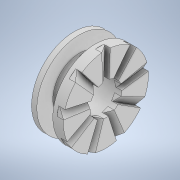
# Autodesk Inventor part: Part11
Saved by Autodesk Inventor 2021 (Build 250183000, 183)
## iProperties
Created: 2022-12-10
Part Number: Part11
Material: Generic
Document SubType Name: Modeling
Designer: user
Density: 1 g/cm^3
Appearance: Default
Author: user
Autodesk Inventor part; units mm, degrees
sketch "Sketch1" plane through (0, 0, 0) normal (0, 0, 1) x (1, 0, 0)
  line L0 (0, 0) -> (0, 40)
  line L1 (0, 40) -> (5, 40)
  line L2 (5, 40) -> (5, 15)
  line L3 (5, 25) -> (20, 25)
  line L4 (20, 15) -> (20, 40)
  line L5 (20, 40) -> (24, 40)
  line L6 (24, 40) -> (24, 0)
  line L7 (24, 0) -> (0, 0)
  line L8 (5, 15) -> (20, 15)
  point P0 (20, 25)
  dimension "d0" = 15
  dimension "d1" = 4
  dimension "d2" = 5
  dimension "d3" = 15
  dimension "d4" = 80
  dimension "d5" = 80
  dimension "d6" = 50
  dimension "d8" = 30
  constraints: 18 end point, 4 perpendicular, 3 horizontal, 2 vertical, 1 point on line
  measures "d0" distance of L3.start L3.end
  measures "d1" distance of L4.end L5.end
  measures "d2" distance of L0.end L1.end
  measures "d3" distance of L4.start L2.end
  measures "d4" diameter of L5 L7
  measures "d5" diameter of L1 L7
  measures "d6" diameter of L3 L7
  measures "d8" diameter of L8 L7
revolve "Revolution1" add sketch "Sketch1" angle 360 about axis through (24, 0, 0) along (-1, 0, 0)
sketch "Sketch2" plane through (0, 0, 0) normal (-1, 0, 0) x (0, 0, 1)
  circle A0 centre (0, 0) radius 15
  point P0 (0, 0)
  dimension "d9" = 30
  constraints: 1 centre point, 1 coincident
  measures "d9" diameter of A0
hole "Hole1" at (0, 0, 0) direction (1, 0, 0) diameter 30 end through all
ref_plane "Work Plane1" through (0, 0, 4) normal (0, 0, 1) x (1, 0, 0)
ref_plane "Work Plane2" through (0, 0, -4) normal (0, 0, 1) x (1, 0, 0)
sketch "Sketch3" plane through (0, 0, 4) normal (0, 0, 1) x (1, 0, 0)
  point P0 (0, 0)
sketch "Sketch6" plane through (24, 0, 0) normal (1, 0, 0) x (0, 0, -1)
  circle A0 centre (0, 0) radius 15 projected
  arc A1 (3, 14.6969) -> (-3, 14.6969) centre (0, 0) ccw
  circle A2 centre (0, 0) radius 40 projected
  arc A3 (4, 39.7995) -> (-4, 39.7995) centre (0, 0) ccw
  line L0 (-3, 14.6969) -> (-4, 39.7995)
  line L1 (4, 39.7995) -> (3, 14.6969)
  line L2 (-11.7451, 9.3301) -> (-28.6468, 27.917)
  arc A4 (-22.5184, 33.0593) -> (-28.6468, 27.917) centre (0, 0) ccw
  line L3 (-22.5184, 33.0593) -> (-7.1489, 13.1869)
  arc A5 (-7.1489, 13.1869) -> (-11.7451, 9.3301) centre (0, 0) ccw
  line L4 (-14.9946, -0.4023) -> (-39.8894, 2.9719)
  arc A6 (-38.5003, 10.8503) -> (-39.8894, 2.9719) centre (0, 0) ccw
  line L5 (-38.5003, 10.8503) -> (-13.9527, 5.5065)
  arc A7 (-13.9527, 5.5065) -> (-14.9946, -0.4023) centre (0, 0) ccw
  line L6 (-11.2279, -9.9465) -> (-32.4674, -23.3639)
  arc A8 (-36.4674, -16.4356) -> (-32.4674, -23.3639) centre (0, 0) ccw
  line L7 (-36.4674, -16.4356) -> (-14.2279, -4.7504)
  arc A9 (-14.2279, -4.7504) -> (-11.2279, -9.9465) centre (0, 0) ccw
  line L8 (-2.2076, -14.8367) -> (-9.8535, -38.7674)
  arc A10 (-17.371, -36.0312) -> (-9.8535, -38.7674) centre (0, 0) ccw
  line L9 (-17.371, -36.0312) -> (-7.8457, -12.7845)
  arc A11 (-7.8457, -12.7845) -> (-2.2076, -14.8367) centre (0, 0) ccw
  line L10 (7.8457, -12.7845) -> (17.371, -36.0312)
  arc A12 (9.8535, -38.7674) -> (17.371, -36.0312) centre (0, 0) ccw
  line L11 (9.8535, -38.7674) -> (2.2076, -14.8367)
  arc A13 (2.2076, -14.8367) -> (7.8457, -12.7845) centre (0, 0) ccw
  line L12 (14.2279, -4.7504) -> (36.4674, -16.4356)
  arc A14 (32.4674, -23.3639) -> (36.4674, -16.4356) centre (0, 0) ccw
  line L13 (32.4674, -23.3639) -> (11.2279, -9.9465)
  arc A15 (11.2279, -9.9465) -> (14.2279, -4.7504) centre (0, 0) ccw
  line L14 (13.9527, 5.5065) -> (38.5003, 10.8503)
  arc A16 (39.8894, 2.9719) -> (38.5003, 10.8503) centre (0, 0) ccw
  line L15 (39.8894, 2.9719) -> (14.9946, -0.4023)
  arc A17 (14.9946, -0.4023) -> (13.9527, 5.5065) centre (0, 0) ccw
  line L16 (7.1489, 13.1869) -> (22.5184, 33.0593)
  arc A18 (28.6468, 27.917) -> (22.5184, 33.0593) centre (0, 0) ccw
  line L17 (28.6468, 27.917) -> (11.7451, 9.3301)
  arc A19 (11.7451, 9.3301) -> (7.1489, 13.1869) centre (0, 0) ccw
  dimension "d30" = 8
  dimension "d31" = 4
  dimension "d32" = 6
  dimension "d33" = 3
  dimension "d36" = 360
  constraints: 41 point on circle, 36 end point, 18 centre point, 10 coincident, 100 other
  measures "d30" distance of L0.end A2.start
  measures "d31" horizontal distance of point (0, 0) A2.start
  measures "d32" distance of L0.start L1.end
  measures "d33" horizontal distance of point (0, 0) L1.end
extrude "Extrusion1" add sketch "Sketch6" along normal blind 6 contours A0 L1 A2 L16
pattern_circular "Circular Pattern2" count 9 over 360 about axis through (115.6547, 0, 0) along (-1, 0, 0) of "Extrusion1"
sketch "Sketch7" plane through (24, 14.6969, -3) normal (0, 0.039805, 0.9992075) x (1, 0, 0)
  point P0 (-24, -14.8047)
sketch "Sketch8" plane through (24, 14.6969, -3) normal (0, 0.039805, 0.9992075) x (1, 0, 0)
  line L0 (0, 25.1225) -> (6, 25.1225) projected
  line L1 (0, 25.1225) -> (1, 25.1225)
  line L2 (1, 25.1225) -> (1, 0.1225)
  line L3 (1, 0.1225) -> (0, 0.1225)
  line L4 (0, 0.1225) -> (0, 25.1225)
  point P0 (-24, -14.8047)
  dimension "d46" = 1
  dimension "d47" = 25
  constraints: 8 end point, 2 parallel, 1 horizontal, 1 perpendicular
  measures "d46" distance of L2.end L3.end
  measures "d47" distance of L1.end L2.end
loft "Loft2" add profiles "Sketch8" section 1 edges at (24, 27.2482, 3.5) (27, 39.7995, 4) (30, 27.2482, 3.5) (27, 14.6969, 3)
pattern_circular "Circular Pattern3" count 9 over 360 about axis through (115.6547, 0, 0) along (-1, 0, 0) of "Loft2"
ref_plane "Work Plane3" through (0, 25, 0) normal (0, 1, 0) x (-1, 0, 0)
sketch "Sketch9" plane through (0, 25, 0) normal (0, 1, 0) x (-1, 0, 0)
  line L0 (-5, 25) -> (-5, -25) projected
  line L1 (-5, 0) -> (-20, 0) construction
  line L2 (-20, 25) -> (-20, -25) projected
  circle A0 centre (-12.5, 0) radius 5
  point P0 (0, 0)
  dimension "d56" = 10
  constraints: 3 midpoint, 2 end point, 1 centre point
  measures "d56" diameter of A0
hole "Hole2" at (12.5, 25, 0) direction (0, -1, 0) diameter 11 depth 12.7625 clearance for "Countersunk Flat Head Screw ISO 2009/7046" size "M10" standard "ISO"
body "Solid1"
